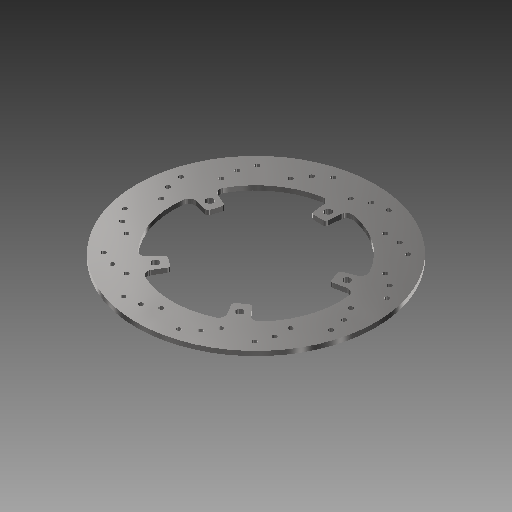
# Autodesk Inventor part: HP2 Raceparts 002
Saved by Autodesk Inventor 2019 (Build 230136000, 136)
## iProperties
Created: 2014-12-15
Part Number: HP2 Raceparts 002
Material: 钢，高强度，低合金
Document SubType Name: Modeling
Designer: Catweazle
Density: 7.85 g/cm^3
Appearance: 钢 - 抛光
Author: Catweazle
Autodesk Inventor part; units mm, degrees
ref_plane "YZ Plane" through (0, 0, 0) normal (1, 0, 0) x (0, 1, 0)
ref_plane "XZ Plane" through (0, 0, 0) normal (0, 1, 0) x (-1, 0, 0)
ref_plane "XY Plane" through (0, 0, 0) normal (0, 0, 1) x (1, 0, 0)
sketch "Skizze1" plane through (0, 0, 0) normal (0, 0, 1) x (1, 0, 0)
  circle A0 centre (0, 0) radius 132.5
  line L0 (-185.5, 0) -> (185.5, 0) projected
  line L1 (0, -185.5) -> (0, 185.5) projected
  circle A1 centre (0, 0) radius 80 construction
  circle A2 centre (0, 80) radius 4
  line L2 (8.2396, 71.7385) -> (9.3594, 84.538)
  line L3 (-8.2396, 71.7385) -> (-9.3594, 84.538)
  line L4 (-5.251, 69) -> (5.251, 69)
  arc A3 (-9.3594, 84.538) -> (-17.4836, 90.8327) centre (-16.3328, 83.9279) ccw
  arc A4 (17.4836, 90.8327) -> (9.3594, 84.538) centre (16.3328, 83.9279) ccw
  arc A5 (-8.2396, 71.7385) -> (-5.251, 69) centre (-5.251, 72) ccw
  arc A6 (5.251, 69) -> (8.2396, 71.7385) centre (5.251, 72) ccw
  circle A7 centre (-76.0845, 24.7214) radius 4
  line L5 (-65.6812, 30.0047) -> (-77.5082, 35.025)
  line L6 (-70.7736, 14.3321) -> (-83.2926, 17.2224)
  line L7 (-67.2455, 16.3282) -> (-64.0002, 26.3162)
  arc A8 (-83.2926, 17.2224) -> (-91.7897, 11.441) centre (-84.8673, 10.4018) ccw
  arc A9 (-80.9843, 44.6967) -> (-77.5082, 35.025) centre (-74.7731, 41.4685) ccw
  arc A10 (-70.7736, 14.3321) -> (-67.2455, 16.3282) centre (-70.0987, 17.2552) ccw
  arc A11 (-64.0002, 26.3162) -> (-65.6812, 30.0047) centre (-66.8534, 27.2432) ccw
  circle A12 centre (-47.0228, -64.7214) radius 4
  line L8 (-48.8328, -53.1946) -> (-57.2621, -62.8914)
  line L9 (-35.5009, -62.8808) -> (-42.1183, -73.894)
  line L10 (-36.309, -58.9086) -> (-44.8053, -52.7357)
  arc A13 (-42.1183, -73.894) -> (-39.2456, -83.7618) centre (-36.1181, -77.4993) ccw
  arc A14 (-67.5346, -63.2086) -> (-57.2621, -62.8914) centre (-62.5451, -58.299) ccw
  arc A15 (-35.5009, -62.8808) -> (-36.309, -58.9086) centre (-38.0724, -61.3357) ccw
  arc A16 (-44.8053, -52.7357) -> (-48.8328, -53.1946) centre (-46.5687, -55.1628) ccw
  circle A17 centre (47.0228, -64.7214) radius 4
  line L11 (35.5009, -62.8808) -> (42.1183, -73.894)
  line L12 (48.8328, -53.1946) -> (57.2621, -62.8914)
  line L13 (44.8053, -52.7357) -> (36.309, -58.9086)
  arc A18 (57.2621, -62.8914) -> (67.5346, -63.2086) centre (62.5451, -58.299) ccw
  arc A19 (39.2456, -83.7618) -> (42.1183, -73.894) centre (36.1181, -77.4993) ccw
  arc A20 (48.8328, -53.1946) -> (44.8053, -52.7357) centre (46.5687, -55.1628) ccw
  arc A21 (36.309, -58.9086) -> (35.5009, -62.8808) centre (38.0724, -61.3357) ccw
  circle A22 centre (76.0845, 24.7214) radius 4
  line L14 (70.7736, 14.3321) -> (83.2926, 17.2224)
  line L15 (65.6812, 30.0047) -> (77.5082, 35.025)
  line L16 (64.0002, 26.3162) -> (67.2455, 16.3282)
  arc A23 (77.5082, 35.025) -> (80.9843, 44.6967) centre (74.7731, 41.4685) ccw
  arc A24 (91.7897, 11.441) -> (83.2926, 17.2224) centre (84.8673, 10.4018) ccw
  arc A25 (65.6812, 30.0047) -> (64.0002, 26.3162) centre (66.8534, 27.2432) ccw
  arc A26 (67.2455, 16.3282) -> (70.7736, 14.3321) centre (70.0987, 17.2552) ccw
  arc A27 (80.9843, 44.6967) -> (17.4836, 90.8327) centre (0, 0) ccw
  arc A28 (-17.4836, 90.8327) -> (-80.9843, 44.6967) centre (0, 0) ccw
  arc A29 (-91.7897, 11.441) -> (-67.5346, -63.2086) centre (0, 0) ccw
  arc A30 (-39.2456, -83.7618) -> (39.2456, -83.7618) centre (0, 0) ccw
  arc A31 (67.5346, -63.2086) -> (91.7897, 11.441) centre (0, 0) ccw
  point P0 (10.0088, 91.9605)
  point P1 (-10.0088, 91.9605)
  point P2 (-8, 69)
  point P3 (8, 69)
  point P4 (-68.095, 13.7137)
  point P5 (-63.1508, 28.9306)
  point P6 (-34.085, -60.5245)
  point P7 (-47.0293, -51.1199)
  point P8 (47.0293, -51.1199)
  point P9 (34.085, -60.5245)
  point P10 (63.1508, 28.9306)
  point P11 (68.095, 13.7137)
  dimension "d2" = 160
  dimension "d0" = 265
  dimension "d3" = 8
  dimension "d5" = 10
  dimension "d6" = 16
  dimension "d7" = 7
  dimension "d8" = 3
  dimension "d11" = 360
  dimension "d36" = 69
  constraints: 50 point on circle, 31 centre point, 30 end point, 23 point on line, 6 tangent, 3 coincident, 2 equal radius, 1 perpendicular, 1 vertical alignment, 119 other
  measures "d0" diameter of A0
  measures "d3" diameter of A2
  measures "d5" angle of L2 L3
  measures "d6" distance of point (-8, 69) point (8, 69)
  measures "d7" radius of A3
  measures "d8" radius of A5
  measures "d36" distance between parallel lines of L0 L4
extrude "Extrusion1" add sketch "Skizze1" against normal blind 5 contours L0 A31 A24 L14 A26 L16 A25 L15 A23 A27 A4 L2 A6 L4 L1 A2 A0 | A0 L1 A30 A19 L11 A21 L13 A20 L12 A18 A31 L0 | L1 A2 L4 A5 L3 A3 A28 A9 L5 A11 L7 A10 L6 A8 A29 L0 A0 | A0 L0 A29 A14 L8 A16 L10 A15 L9 A13 A30 L1
sketch "Skizze2" plane through (0, 0, 0) normal (0, 0, 1) x (1, 0, 0)
  line L0 (-185.5, 0) -> (185.5, 0) construction
  line L1 (0, -185.5) -> (0, 185.5) construction
  circle A0 centre (0, 105) radius 2.5
  circle A1 centre (15, 112.5) radius 2.5
  circle A2 centre (32, 115) radius 2.5
  dimension "d23" = 5
  dimension "d24" = 5
  dimension "d25" = 5
  dimension "d26" = 105
  dimension "d27" = 112.5
  dimension "d28" = 115
  dimension "d29" = 15
  dimension "d30" = 32
  constraints: 3 centre point, 1 point on line
  measures "d23" diameter of A0
  measures "d24" diameter of A1
  measures "d25" diameter of A2
  measures "d26" distance from line of L0 A0.centre
  measures "d27" distance from line of L0 A1.centre
  measures "d28" distance from line of L0 A2.centre
  measures "d29" distance from line of L1 A1.centre
  measures "d30" distance from line of L1 A2.centre
extrude "Extrusion2" cut sketch "Skizze2" against normal through all
pattern_circular "Runde Anordnung1" count 12 over 360 about axis through (0, 0, -10) along (0, 0, 1) of "Extrusion2"
